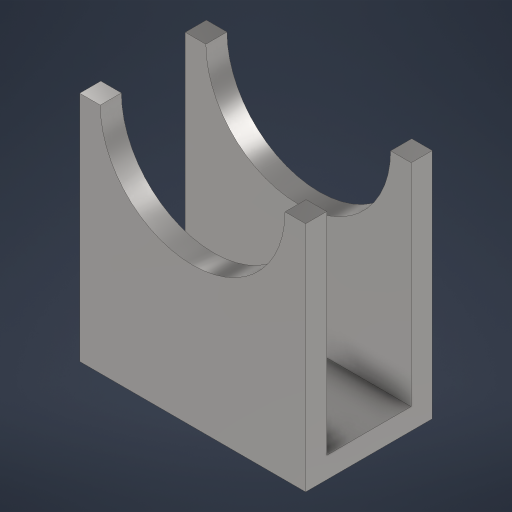
# Autodesk Inventor part: Support
Saved by Autodesk Inventor 2023 (Build 270158000, 158)
## iProperties
Created: 2022-08-20
Part Number: Support
Material: Stainless Steel
Document SubType Name: Modeling
Designer: Mike
Density: 8 g/cm^3
Appearance: Semi-Polished
Author: Mike
Autodesk Inventor part; units mm, degrees
ref_plane "YZ Plane" through (0, 0, 0) normal (1, 0, 0) x (0, 1, 0)
ref_plane "XZ Plane" through (0, 0, 0) normal (0, 1, 0) x (-1, 0, 0)
sketch "Sketch1" plane through (0, 0, 0) normal (0, 0, 1) x (1, 0, 0)
  arc A0 (-87.5, 0) -> (87.5, 0) centre (0, 0) ccw
  line L0 (-87.5, 0) -> (87.5, 0) construction
  line L1 (-87.5, -200) -> (87.5, -200)
  line L2 (-87.5, -220) -> (87.5, -220)
  line L3 (-87.5, 0) -> (-107.5, 0)
  line L4 (0, 0) -> (-107, 0)
  line L5 (-107, 0) -> (-107, -200)
  line L6 (-107, -200) -> (-87.5, -200)
  line L7 (-107, -200) -> (-107, -220)
  line L8 (-107, -220) -> (-87.5, -220)
  line L9 (0, 0) -> (107, 0)
  line L10 (107, 0) -> (107, -220)
  line L11 (107, -220) -> (87.5, -220)
  line L12 (87.5, -200) -> (107, -200)
  point P0 (87.5, 0)
  dimension "d0" = 175
  dimension "d1" = 200
  dimension "d9" = 107
  dimension "d10" = 107
  dimension "d13" = 90
  dimension "d15" = 200
  dimension "d17" = 200
  dimension "d18" = 214.5
  dimension "d21" = 20
  constraints: 26 end point, 6 perpendicular, 3 horizontal, 2 point on circle, 2 point on line, 1 centre point, 1 coincident, 1 vertical
  measures "d0" diameter of A0
  measures "d1" distance of L0.start L1.start
  measures "d9" distance of L4.start L4.end
  measures "d10" distance of L4.start L9.end
  measures "d13" angle of L10 L4
  measures "d15" distance between parallel lines of L12 L9
  measures "d17" distance between parallel lines of L6 L4
  measures "d18" distance from line of L3.end L10
  measures "d21" distance between parallel lines of L2 L1
extrude "Extrusion1" add sketch "Sketch1" along normal blind 20 contours A0 L9 L10 L12 L1 L6 L5 L3
extrude "Extrusion2" add sketch "Sketch1" along normal blind 20 and the other way blind 100 contours L6 L1 L12 L10 L11 L2 L8 L7
ref_plane "Work Plane1" through (0, 0, -40) normal (0, 0, -1) x (1, 0, 0)
mirror "Mirror1" about plane through (0, 0, -40) normal (0, 0, -1) of "Extrusion1"
body "Solid1"
